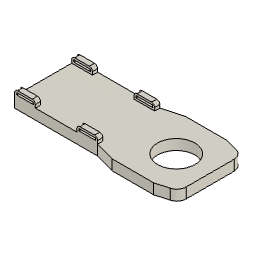
proto (Autodesk Fusion 360 design; units mm, degrees)
Autodesk Fusion 360 part; units mm, degrees
sketch "Sketch1" plane through (0, 0, 0) normal (0, 0, 1) x (1, 0, 0)
  line L0 (0, 0) -> (101.6, 0)
  line L1 (101.6, 0) -> (101.6, -76.2)
  line L2 (101.6, -76.2) -> (0, -76.2)
  line L3 (0, -76.2) -> (0, 0)
  line L4 (101.6, 0) -> (126.0466, 6.8938)
  line L5 (126.0466, 6.8938) -> (176.8466, 6.8938)
  line L6 (176.8466, 6.8938) -> (201.2932, 0)
  line L7 (201.2932, 0) -> (201.2932, -76.2)
  line L8 (201.2932, -76.2) -> (176.8466, -82.9718)
  line L9 (176.8466, -82.9718) -> (126.0466, -82.9718)
  line L10 (126.0466, -82.9718) -> (101.6, -76.2)
  dimension "d1" = 101.6
  dimension "d2" = 76.2
  dimension "d3" = 25.4
  dimension "d4" = 50.8
  dimension "d5" = 25.4
  constraint horizontal L0
  constraint vertical L1
  constraint horizontal L2
  constraint vertical L3
  constraint coincident L0.start L3.end
  constraint perpendicular L1 L5
  constraint perpendicular L5 L7
  constraint parallel L5 L9
  measures "d1" distance of L0.start L0.end
  measures "d2" distance of L0.start L2.end
  measures "d3" distance of L0.end L4.end
  measures "d4" distance of L4.end L5.end
  measures "d5" distance of L5.end L6.end
extrude "Extrude1" add sketch "Sketch1" along normal blind 12.7
fillet "Fillet1" radius 11.43 2 edges at (201.2932, -76.2, 6.35) (201.2932, 0, 6.35)
sketch "Sketch2" plane through (0, 0, 12.7) normal (0, 0, 1) x (-1, 0, 0)
  arc A0 (-201.2932, 8.6526) -> (-192.9654, -2.3484) centre (-189.8632, 8.6526) ccw
  line L0 (-192.9654, -2.3484) -> (-176.8466, -6.8938)
  line L1 (-176.8466, -6.8938) -> (-126.0466, -6.8938)
  line L2 (-126.0466, -6.8938) -> (-101.6, 0)
  line L3 (-101.6, 0) -> (0, 0)
  line L4 (0, 0) -> (0, 76.2)
  line L5 (0, 76.2) -> (-101.6, 76.2)
  line L6 (-101.6, 76.2) -> (-126.0466, 82.9718)
  line L7 (-126.0466, 82.9718) -> (-176.8466, 82.9718)
  line L8 (-176.8466, 82.9718) -> (-192.9144, 78.5209)
  arc A1 (-192.9144, 78.5209) -> (-201.2932, 67.5057) centre (-189.8632, 67.5057) ccw
  line L9 (-201.2932, 67.5057) -> (-201.2932, 8.6526)
  line L10 (0, 0) -> (-25.4, 0)
  line L11 (-25.4, 0) -> (-25.4, 6.35)
  line L12 (-25.4, 6.35) -> (0, 6.35)
  line L13 (0, 6.35) -> (0, 0)
  line L14 (0, 38.1) -> (-145.8184, 38.1) construction
  line L15 (-50.8, 0) -> (-50.8, 76.2) construction
  line L16 (0, 76.2) -> (-25.4, 76.2)
  line L17 (0, 69.85) -> (0, 76.2)
  line L18 (-25.4, 69.85) -> (0, 69.85)
  line L19 (-25.4, 76.2) -> (-25.4, 69.85)
  line L20 (-76.2, 0) -> (-76.2, 6.35)
  line L21 (-101.6, 0) -> (-76.2, 0)
  line L22 (-101.6, 6.35) -> (-101.6, 0)
  line L23 (-76.2, 6.35) -> (-101.6, 6.35)
  line L24 (-76.2, 69.85) -> (-101.6, 69.85)
  line L25 (-101.6, 69.85) -> (-101.6, 76.2)
  line L26 (-101.6, 76.2) -> (-76.2, 76.2)
  line L27 (-76.2, 76.2) -> (-76.2, 69.85)
  dimension "d10" = 25.4
  dimension "d11" = 6.35
  constraint horizontal L10
  constraint vertical L11
  constraint horizontal L12
  constraint vertical L13
  constraint coincident L3.end L4.start
  constraint midpoint L4 L14.start
  constraint perpendicular L4 L14
  constraint midpoint L3 L15.start
  constraint midpoint L5 L15.end
  constraint symmetric L3.end L14 L4.end
  constraint symmetric L10.end L14 L16.end
  constraint symmetric L11.end L14 L18.start
  constraint symmetric L12.end L14 L17.start
  constraint symmetric L3.end L15 L2.end
  constraint symmetric L10.end L15 L20.start
  constraint symmetric L11.end L15 L20.end
  constraint symmetric L12.end L15 L22.start
  constraint symmetric L15 L4.end L5.end
  constraint symmetric L15 L16.end L26.end
  constraint symmetric L15 L17.start L24.end
  constraint symmetric L15 L18.start L24.start
  measures "d10" distance of L3.end L10.end
  measures "d11" distance of L3.end L12.end
extrude "Extrude2" add sketch "Sketch2" along normal blind 7.62 contours L3 L20 L21 L22 L23 | L5 L24 L25 L26 L27 | L3 L4 L10 L11 L12 L13 | L4 L5 L16 L17 L18 L19
sketch "Sketch3" plane through (0, -76.2, 0) normal (0, -1, 0) x (1, 0, 0)
  line L0 (0, 0) -> (101.6, 0)
  line L1 (101.6, 0) -> (101.6, 12.7)
  line L2 (101.6, 12.7) -> (101.6, 20.32)
  line L3 (101.6, 20.32) -> (76.2, 20.32)
  line L4 (76.2, 20.32) -> (76.2, 12.7)
  line L5 (76.2, 12.7) -> (25.4, 12.7)
  line L6 (25.4, 12.7) -> (25.4, 20.32)
  line L7 (25.4, 20.32) -> (0, 20.32)
  line L8 (0, 20.32) -> (0, 0)
  line L9 (2.54, 17.78) -> (22.86, 17.78)
  line L10 (22.86, 17.78) -> (22.86, 15.24)
  line L11 (22.86, 15.24) -> (2.54, 15.24)
  line L12 (2.54, 15.24) -> (2.54, 17.78)
  line L13 (78.74, 17.78) -> (99.06, 17.78)
  line L14 (99.06, 17.78) -> (99.06, 15.24)
  line L15 (99.06, 15.24) -> (78.74, 15.24)
  line L16 (78.74, 15.24) -> (78.74, 17.78)
  constraint horizontal L9
  constraint vertical L10
  constraint horizontal L11
  constraint vertical L12
  constraint horizontal L13
  constraint vertical L14
  constraint horizontal L15
  constraint vertical L16
extrude "Extrude3" cut sketch "Sketch3" against normal blind 86.36 contours L9 L10 L11 L12 | L13 L14 L15 L16
fillet "Fillet2" radius 3.81 8 edges at (101.6, -3.175, 20.32) (76.2, -3.175, 20.32) (101.6, -73.025, 20.32) (76.2, -73.025, 20.32) (25.4, -73.025, 20.32) (0, -73.025, 20.32) (0, -3.175, 20.32) (25.4, -3.175, 20.32)
sketch "Sketch4" plane through (0, 0, 12.7) normal (0, 0, 1) x (-1, 0, 0)
  line L0 (-101.6, 0) -> (-101.6, 6.35)
  line L1 (-101.6, 6.35) -> (-76.2, 6.35)
  line L2 (-76.2, 6.35) -> (-76.2, 0)
  line L3 (-76.2, 0) -> (-25.4, 0)
  line L4 (-25.4, 0) -> (-25.4, 6.35)
  line L5 (-25.4, 6.35) -> (0, 6.35)
  line L6 (0, 6.35) -> (0, 69.85)
  line L7 (0, 69.85) -> (-25.4, 69.85)
  line L8 (-25.4, 69.85) -> (-25.4, 76.2)
  line L9 (-25.4, 76.2) -> (-76.2, 76.2)
  line L10 (-76.2, 76.2) -> (-76.2, 69.85)
  line L11 (-76.2, 69.85) -> (-101.6, 69.85)
  line L12 (-101.6, 69.85) -> (-101.6, 76.2)
  line L13 (-101.6, 76.2) -> (-126.0466, 82.9718)
  line L14 (-126.0466, 82.9718) -> (-176.8466, 82.9718)
  line L15 (-176.8466, 82.9718) -> (-192.9144, 78.5209)
  arc A0 (-192.9144, 78.5209) -> (-201.2932, 67.5057) centre (-189.8632, 67.5057) ccw
  line L16 (-201.2932, 67.5057) -> (-201.2932, 8.6526)
  arc A1 (-201.2932, 8.6526) -> (-192.9654, -2.3484) centre (-189.8632, 8.6526) ccw
  line L17 (-192.9654, -2.3484) -> (-176.8466, -6.8938)
  line L18 (-176.8466, -6.8938) -> (-126.0466, -6.8938)
  line L19 (-126.0466, -6.8938) -> (-101.6, 0)
  circle A2 centre (-160.0534, 38.3696) radius 22.86
  dimension "d18" = 45.72
  measures "d18" diameter of A2
extrude "Extrude4" cut sketch "Sketch4" against normal blind 38.1 contours A2
